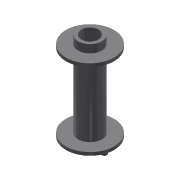
# Autodesk Inventor part: bobbin
Saved by Autodesk Inventor 2022 (Build 260148000, 148)
## iProperties
Shininess: 64.0
Length Units: 11272
Angle Units: 11279
Time Units: 11290
Mass Units: 11286
Length Display Precision: 3
Angle Display Precision: 2
Created: 2002-05-01
Part Number: bobbin
Material: Delrin, Black
Document SubType Name: Modeling
Designer: Administrator
Density: 1.425 g/cm^3
Appearance: Smooth - Medium Gray
Density: 1.4249999999999998
Volumn: 1.8073874128000593
Area: 29.882755635617393
PropertySet Name: Model Information
Control State: 0
Master: False
Checked Out: False
Author: Administrator
Autodesk Inventor part; units mm, degrees
ref_plane "YZ Plane" through (0, 0, 0) normal (1, 0, 0) x (0, 1, 0)
ref_plane "XZ Plane" through (0, 0, 0) normal (0, 1, 0) x (-1, 0, 0)
ref_plane "XY Plane" through (0, 0, 0) normal (0, 0, 1) x (1, 0, 0)
sketch "Sketch1" plane through (0, 0, 0) normal (0, 0, 1) x (1, 0, 0)
  line L0 (-10.9402, 26.9819) -> (-10.9402, -11.1181)
  line L1 (-10.9402, -11.1181) -> (-9.6702, -11.1181)
  line L2 (-9.6702, -11.1181) -> (-9.6702, -7.9431)
  line L3 (-9.6702, -7.9431) -> (-4.8442, -7.9431)
  line L4 (-4.8442, -7.9431) -> (-4.8442, -6.6731)
  line L5 (-4.8442, -6.6731) -> (-9.6702, -6.6731)
  line L6 (-9.6702, -6.6731) -> (-9.6702, 22.5369)
  line L7 (-9.6702, 22.5369) -> (-4.8442, 22.5369)
  line L8 (-4.8442, 22.5369) -> (-4.8442, 23.8069)
  line L9 (-4.8442, 23.8069) -> (-9.6702, 23.8069)
  line L10 (-9.6702, 23.8069) -> (-9.6702, 26.9819)
  line L11 (-9.6702, 26.9819) -> (-10.9402, 26.9819)
  line L12 (-14.3692, 26.9819) -> (-14.3692, -11.1181) construction
  dimension "d0" = 9.525
  dimension "d1" = 4.699
  dimension "d2" = 38.1
  dimension "d3" = 3.175
  dimension "d4" = 1.27
  dimension "d5" = 1.27
  constraints: 26 end point, 10 parallel, 5 collinear, 2 horizontal alignment, 2 perpendicular, 1 vertical
  measures "d0" horizontal distance of L8.end L12.start
  measures "d1" distance of L10.end L12.start
  measures "d2" distance of L0.end L0.start
  measures "d3" distance of L9.end L10.end
  measures "d4" distance of L7.end L8.end
  measures "d5" distance of L10.end L0.start
revolve "Revolution1" add sketch "Sketch1" angle 360 about axis through (-14.3692, 26.9819, 0) along (0, -1, 0)
sketch "Sketch2" plane through (-14.3692, 23.8069, 0) normal (0, 1, 0) x (1, 0, 0)
  circle A0 centre (0, 0) radius 9.525 projected
  point P0 (-5.715, 0)
  dimension "d18" = 5.715
  constraints: 1 horizontal alignment
  measures "d18" distance of A0.centre point (-5.715, 0)
hole "Hole1" at (-20.0842, 23.8069, 0) direction (0, -1, 0) diameter 1.5875 end up to surface
sketch "Sketch3" plane through (-14.3692, -7.9431, 0) normal (0, -1, 0) x (1, 0, 0)
  circle A0 centre (0, 0) radius 4.699 projected
  line L0 (4.5878, 1.016) -> (5.715, 1.016)
  arc A1 (5.715, -1.016) -> (5.715, 1.016) centre (5.715, 0) ccw
  line L1 (5.715, -1.016) -> (4.5878, -1.016)
  dimension "d26" = 2.032
  dimension "d27" = 5.715
  constraints: 4 end point, 4 point on circle, 2 tangent, 1 centre point, 1 horizontal, 1 horizontal alignment, 1 parallel
  measures "d26" distance of L0.end L1.start
  measures "d27" distance of A1.centre A0.centre
extrude "Extrusion1" add sketch "Sketch3" along normal up to surface (3.175 mm away) contours A0 L0 A1 L1
body "Solid1"
